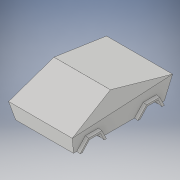
# Autodesk Inventor part: tesla cyber truck
Saved by Autodesk Inventor 2018 (Build 220112000, 112)
## iProperties
Created: 2020-01-07
Part Number: tesla cyber truck
Material: Generic
Document SubType Name: Modeling
Designer: AOFUser
Density: 1 g/cm^3
Appearance: Default
Author: AOFUser
Autodesk Inventor part; units mm, degrees
ref_plane "YZ Plane" through (0, 0, 0) normal (1, 0, 0) x (0, 1, 0)
ref_plane "XZ Plane" through (0, 0, 0) normal (0, 1, 0) x (-1, 0, 0)
ref_plane "XY Plane" through (0, 0, 0) normal (0, 0, 1) x (1, 0, 0)
sketch "Sketch1" plane through (0, 0, 0) normal (0, 1, 0) x (-1, 0, 0)
  line L0 (0, 0) -> (-50.8, 0)
  line L1 (-50.8, 0) -> (-50.8, -76.2)
  line L2 (-50.8, -76.2) -> (0, -76.2)
  line L3 (0, -76.2) -> (0, 0)
  dimension "d0" = 50.8
  dimension "d1" = 76.2
  constraints: 8 end point, 2 parallel, 1 horizontal, 1 perpendicular
  measures "d0" distance of L2.end L1.end
  measures "d1" distance of L1.end L0.end
extrude "Extrusion1" add sketch "Sketch1" along normal blind 17.78
chamfer "Chamfer1" distance 17.78 distance2 3.175 1 edges at (50.8, 0, -38.1) measured on face at (50.8, 0.5, -38.1)
chamfer "Chamfer2" distance 17.78 distance2 3.175 1 edges at (0, 0, -38.1) measured on face at (0, 0.5, -38.1)
chamfer "Chamfer3" distance 17.78 distance2 3.175 1 edges at (25.4, 0, -76.2) measured on face at (25.4, 0.5, -76.2)
chamfer "Chamfer4" distance 12.7 distance2 3.175 1 edges at (25.4, 0, 0) measured on face at (25.4, 0.5, 0)
sketch "Sketch2" plane through (49.8929, 12.7, 0) normal (0.9844276, -0.1757906, 0) x (0, 0, -1)
  line L0 (3.175, -12.9009) -> (73.025, -12.9009) projected
  line L1 (3.175, -12.9009) -> (5.715, -12.9009)
  line L2 (5.715, -12.9009) -> (26.035, -12.9009)
  line L3 (26.035, -12.9009) -> (20.955, -4.1021)
  line L4 (20.955, -4.1021) -> (10.795, -4.1021)
  line L5 (10.795, -4.1021) -> (5.715, -12.9009)
  line L6 (73.025, -12.9009) -> (73.025, -20.7148) projected
  line L7 (73.025, -12.9009) -> (70.485, -12.9009)
  line L8 (70.485, -12.9009) -> (50.165, -12.9009)
  line L9 (50.165, -12.9009) -> (55.245, -4.1021)
  line L10 (55.245, -4.1021) -> (65.405, -4.1021)
  line L11 (65.405, -4.1021) -> (70.485, -12.9009)
  point P0 (0, -21.2729)
  dimension "d16" = 2.54
  dimension "d17" = 20.32
  dimension "d18" = 10.16
  dimension "d19" = 60
  dimension "d20" = 10.16
  dimension "d21" = 2.54
  dimension "d22" = 20.32
  dimension "d23" = 10.16
  dimension "d24" = 60
  dimension "d25" = 10.16
  constraints: 20 end point, 5 point on line, 2 parallel
  measures "d16" distance of L0.start L1.end
  measures "d17" distance of L1.end L2.end
  measures "d18" distance of L2.end L3.end
  measures "d19" angle of L3 L2
  measures "d20" distance of L3.end L4.end
  measures "d21" distance of L0.end L7.end
  measures "d22" distance of L7.end L8.end
  measures "d23" distance of L8.end L9.end
  measures "d24" angle of L8 L9
  measures "d25" distance of L9.end L10.end
extrude "Extrusion2" add sketch "Sketch2" along normal blind 2.54
sketch "Sketch3" plane through (0.9071, 12.7, -76.2) normal (-0.9844276, -0.1757906, 0) x (0, 0, 1)
  line L0 (3.175, -20.7148) -> (3.175, -12.9009) projected
  line L1 (3.175, -12.9009) -> (5.715, -12.9009)
  line L2 (3.175, -12.9009) -> (73.025, -12.9009) projected
  line L3 (5.715, -12.9009) -> (26.035, -12.9009)
  line L4 (5.715, -12.9009) -> (10.795, -4.1021)
  line L5 (5.715, -12.9009) -> (15.875, -12.9009) construction
  line L6 (10.795, -4.1021) -> (20.955, -4.1021)
  line L7 (20.955, -4.1021) -> (26.035, -12.9009)
  line L8 (73.025, -12.9009) -> (73.025, -20.7148) projected
  line L9 (73.025, -12.9009) -> (70.485, -12.9009)
  line L10 (70.485, -12.9009) -> (50.165, -12.9009)
  line L11 (50.165, -12.9009) -> (55.245, -4.1021)
  line L12 (55.245, -4.1021) -> (65.405, -4.1021)
  line L13 (65.405, -4.1021) -> (70.485, -12.9009)
  point P0 (76.2, -12.3428)
  dimension "d28" = 2.54
  dimension "d29" = 20.32
  dimension "d30" = 10.16
  dimension "d31" = 60
  dimension "d32" = 10.16
  dimension "d33" = 2.54
  dimension "d34" = 20.32
  dimension "d35" = 10.16
  dimension "d36" = 60
  dimension "d37" = 10.16
  constraints: 22 end point, 5 point on line, 2 horizontal, 1 equal length, 1 parallel
  measures "d28" distance of L0.end L1.end
  measures "d29" distance of L1.end L3.end
  measures "d30" distance of L1.end L4.end
  measures "d31" angle of L5 L4
  measures "d32" distance of L4.end L6.end
  measures "d33" distance of L2.end L9.end
  measures "d34" distance of L9.end L10.end
  measures "d35" distance of L10.end L11.end
  measures "d36" angle of L10 L11
  measures "d37" distance of L11.end L12.end
extrude "Extrusion3" add sketch "Sketch3" along normal blind 2.54
sketch "Sketch4" plane through (-1.5933, 12.2535, -76.2) normal (-0.9844276, -0.1757906, 0) x (0, 0, 1)
  line L0 (5.715, -12.9009) -> (26.035, -12.9009) projected
  line L1 (5.715, -12.9009) -> (15.875, -12.9009)
  line L2 (5.715, -12.9009) -> (7.493, -12.9009)
  line L3 (7.493, -12.9009) -> (11.684, -5.6419)
  line L4 (11.684, -5.6419) -> (20.066, -5.6419)
  line L5 (20.066, -5.6419) -> (24.257, -12.9009)
  line L6 (24.257, -12.9009) -> (20.066, -20.1599)
  line L7 (20.066, -20.1599) -> (11.684, -20.1599)
  line L8 (11.684, -20.1599) -> (7.493, -12.9009)
  line L9 (50.165, -12.9009) -> (60.325, -12.9009)
  line L10 (50.165, -12.9009) -> (70.485, -12.9009) projected
  line L11 (50.165, -12.9009) -> (51.943, -12.9009)
  line L12 (51.943, -12.9009) -> (56.134, -5.6419)
  line L13 (56.134, -5.6419) -> (64.516, -5.6419)
  line L14 (64.516, -5.6419) -> (68.707, -12.9009)
  line L15 (68.707, -12.9009) -> (64.516, -20.1599)
  line L16 (64.516, -20.1599) -> (56.134, -20.1599)
  line L17 (56.134, -20.1599) -> (51.943, -12.9009)
  point P0 (76.2, -12.3428)
  dimension "d40" = 10.16
  dimension "d41" = 1.778
  dimension "d42" = 10.16
  dimension "d43" = 1.778
  constraints: 32 end point, 2 coincident, 2 midpoint, 2 point on line, 26 other
  measures "d40" distance of L0.start L1.end
  measures "d41" distance of L0.start L2.end
  measures "d42" distance of L9.start L9.end
  measures "d43" distance of L9.start L11.end
extrude "Extrusion4" cut sketch "Sketch4" against normal blind 7.62
sketch "Sketch5" plane through (52.3933, 12.2535, 0) normal (0.9844276, -0.1757906, 0) x (0, 0, -1)
  line L0 (5.715, -12.9009) -> (26.035, -12.9009) projected
  line L1 (5.715, -12.9009) -> (15.875, -12.9009)
  line L2 (5.715, -12.9009) -> (7.493, -12.9009)
  line L3 (7.493, -12.9009) -> (11.684, -5.6419)
  line L4 (11.684, -5.6419) -> (20.066, -5.6419)
  line L5 (20.066, -5.6419) -> (24.257, -12.9009)
  line L6 (24.257, -12.9009) -> (20.066, -20.1599)
  line L7 (20.066, -20.1599) -> (11.684, -20.1599)
  line L8 (11.684, -20.1599) -> (7.493, -12.9009)
  line L9 (50.165, -12.9009) -> (70.485, -12.9009) projected
  line L10 (50.165, -12.9009) -> (60.325, -12.9009)
  line L11 (50.165, -12.9009) -> (51.943, -12.9009)
  line L12 (51.943, -12.9009) -> (56.134, -5.6419)
  line L13 (56.134, -5.6419) -> (64.516, -5.6419)
  line L14 (64.516, -5.6419) -> (68.707, -12.9009)
  line L15 (68.707, -12.9009) -> (64.516, -20.1599)
  line L16 (64.516, -20.1599) -> (56.134, -20.1599)
  line L17 (56.134, -20.1599) -> (51.943, -12.9009)
  point P0 (0, -21.2729)
  dimension "d46" = 10.16
  dimension "d47" = 1.778
  dimension "d48" = 10.16
  dimension "d49" = 1.778
  constraints: 32 end point, 2 coincident, 2 midpoint, 2 point on line, 26 other
  measures "d46" distance of L0.start L1.end
  measures "d47" distance of L0.start L2.end
  measures "d48" distance of L9.start L10.end
  measures "d49" distance of L9.start L11.end
extrude "Extrusion5" cut sketch "Sketch5" against normal blind 7.62
chamfer "Chamfer9" distance 76.2 distance2 5.08 3 edges at (50.8, 17.7799, 0) (0, 17.7799, 0) (25.4, 17.78, 0) measured on face at (50.8, 17.78, -25.4) measured on face at (25.4, 17.78, -0.5) measured on face at (0, 17.78, -50.8)
sketch "Sketch9" plane through (0, 17.78, -76.2) normal (0, 0.9977852, 0.066519) x (1, 0, 0)
  line L0 (0.9071, -76.3691) -> (3.175, -74.046) projected
  line L1 (0.9071, -76.3691) -> (0, 0)
  line L2 (49.8929, -76.3691) -> (50.8, 0) projected
  line L3 (0, 0) -> (50.8, 0)
  line L4 (50.8, 0) -> (49.8929, -76.3691)
  line L5 (49.8929, -76.3691) -> (0.9071, -76.3691)
  point P0 (0, -77.2139)
  constraints: 8 end point, 1 collinear, 1 horizontal, 1 parallel
extrude "Extrusion7" add sketch "Sketch9" along normal blind 12.7
chamfer "Chamfer10" distance 3.175 distance2 12.7 1 edges at (50.3464, 27.9119, -37.2552) measured on face at (49.8465, 27.9123, -37.2611)
chamfer "Chamfer11" distance 3.175 distance2 12.7 1 edges at (0.4536, 27.9119, -37.2552) measured on face at (0.9535, 27.9123, -37.2611)
chamfer "Chamfer12" distance 33.02 distance2 12.7 1 edges at (25.4, 25.3719, 0.8448) measured on face at (25.4, 25.4051, 0.3459)
chamfer "Chamfer13" distance 43.3324 distance2 12.7 1 edges at (25.4, 30.4519, -75.3552) measured on face at (25.4, 30.4186, -74.8563)
sketch "Sketch12" plane through (5.908, 13.593, -76.2) normal (-0.9844276, -0.1757906, 0) x (0, 0, 1)
  line L0 (23.7333, -13.808) -> (8.0167, -13.808) projected
  line L1 (15.875, -13.808) -> (15.875, -9.617)
  circle A0 centre (15.875, -9.617) radius 1.27
  line L2 (68.1833, -13.808) -> (52.4667, -13.808) projected
  line L3 (60.325, -13.808) -> (60.325, -9.617)
  circle A1 centre (60.325, -9.617) radius 1.27
  point P0 (76.2, -12.3428)
  dimension "d87" = 4.191
  dimension "d88" = 2.54
  dimension "d89" = 4.191
  dimension "d90" = 2.54
  constraints: 4 end point, 2 centre point, 2 coincident, 2 midpoint, 2 vertical
  measures "d87" distance of L1.start L1.end
  measures "d88" diameter of A0
  measures "d89" distance of L3.start L3.end
  measures "d90" diameter of A1
extrude "Extrusion8" cut sketch "Sketch12" against normal blind 12.7
sketch "Sketch13" plane through (44.892, 13.593, 0) normal (0.9844276, -0.1757906, 0) x (0, 0, -1)
  line L0 (23.7333, -13.808) -> (8.0167, -13.808) projected
  line L1 (15.875, -13.808) -> (15.875, -9.617)
  line L2 (68.1833, -13.808) -> (52.4667, -13.808) projected
  line L3 (60.325, -13.808) -> (60.325, -9.617)
  circle A0 centre (15.875, -9.617) radius 1.27
  circle A1 centre (60.325, -9.617) radius 1.27
  point P0 (0, -21.2729)
  dimension "d93" = 4.191
  dimension "d94" = 4.191
  dimension "d95" = 2.54
  dimension "d96" = 2.54
  constraints: 4 end point, 2 centre point, 2 coincident, 2 midpoint, 2 vertical
  measures "d93" distance of L1.start L1.end
  measures "d94" distance of L3.start L3.end
  measures "d95" diameter of A0
  measures "d96" diameter of A1
extrude "Extrusion9" cut sketch "Sketch13" against normal blind 12.7
body "Solid1"
